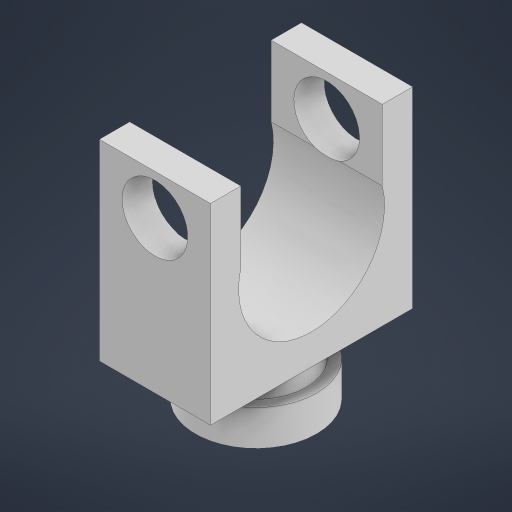
# Autodesk Inventor part: Part5
Saved by Autodesk Inventor 2023 (Build 270158030, 158C)
## iProperties
Created: 2023-02-06
Part Number: Part5
Material: Generic
Document SubType Name: Modeling
Designer: Monster
Density: 1 g/cm^3
Appearance: Default
Author: Monster
Autodesk Inventor part; units mm, degrees
ref_plane "YZ Plane" through (0, 0, 0) normal (1, 0, 0) x (0, 1, 0)
ref_plane "XZ Plane" through (0, 0, 0) normal (0, 1, 0) x (-1, 0, 0)
ref_plane "XY Plane" through (0, 0, 0) normal (0, 0, 1) x (1, 0, 0)
sketch "Sketch2" plane through (0, 0, 0) normal (0, 1, 0) x (-1, 0, 0)
  line L0 (0, 0) -> (0, -20)
  line L1 (0, -20) -> (11, -20)
  line L2 (11, -20) -> (11, 0)
  line L3 (11, 0) -> (0, 0)
  dimension "d3" = 11
  dimension "d35" = 20
  constraints: 8 end point, 3 perpendicular, 1 vertical
  measures "d3" distance of L0.end L1.end
  measures "d35" distance between parallel lines of L3 L1
extrude "Extrusion1" add sketch "Sketch2" along normal blind 15
sketch "Sketch3" plane through (-11, 0, 0) normal (0, 0, 1) x (1, 0, 0)
  line L0 (0, 0) -> (11, 0) projected
  line L1 (11, 0) -> (11, 15) projected
  line L2 (0, 15) -> (11, 15) projected
  line L3 (0, 0) -> (0, 15) projected
  line L4 (11, 15) -> (0, 15) projected
  circle A0 centre (5.5, 15) radius 3.25
  line L5 (0, 15) -> (0, 19)
  line L6 (0, 19) -> (11, 19)
  line L7 (11, 19) -> (11, 15)
  point P0 (8.75, 15)
  point P1 (2.25, 15)
  dimension "d33" = 6.5
  dimension "d34" = 4
  constraints: 6 end point, 2 perpendicular, 1 centre point, 1 midpoint, 1 vertical
  measures "d33" diameter of A0
  measures "d34" distance between parallel lines of L2 L6
extrude "Extrusion2" cut sketch "Sketch3" against normal blind 32.25 contours L2 A0 picked at (4.4481, 14.7407)
sketch "Sketch4" plane through (0, 0, 0) normal (1, 0, 0) x (0, 0, -1)
  line L0 (0, 0) -> (20, 0) projected
  line L1 (20, 0) -> (20, 15) projected
  line L2 (0, 15) -> (20, 15) projected
  line L3 (0, 0) -> (0, 15) projected
  line L4 (0, 15) -> (3, 15)
  line L5 (0, 15) -> (20, 15) projected
  line L6 (20, 15) -> (17, 15)
  line L7 (17, 15) -> (17, 12)
  line L8 (0, 11.75) -> (20, 11.75) projected
  line L9 (17, 12) -> (3, 12)
  line L10 (3, 12) -> (3, 15)
  line L11 (20, 0) -> (0, 0) projected
  line L12 (10, 0) -> (10, 3)
  arc A0 (3, 12) -> (17, 12) centre (10, 10.2222) ccw
  line L13 (3, 15) -> (3, 23.7535)
  line L14 (3, 23.7535) -> (17, 23.7535)
  line L15 (17, 23.7535) -> (17, 15)
  point P0 (17, 15)
  dimension "d11" = 3
  dimension "d12" = 3
  dimension "d36" = 3
  dimension "d37" = 3
  constraints: 18 end point, 5 perpendicular, 3 point on circle, 2 point on line, 2 vertical, 1 centre point, 1 midpoint
  measures "d11" distance of L6.end L7.end
  measures "d12" distance of L12.start L12.end
  measures "d36" distance between parallel lines of L3 L10
  measures "d37" distance between parallel lines of L1 L7
extrude "Extrusion3" cut sketch "Sketch4" against normal blind 32.25 contours A0 L8 | A0 L9 L8 | L2 L7 L9 L10
sketch "Sketch7" plane through (0, 0, 0) normal (0, -1, 0) x (1, 0, 0)
  line L0 (0, -20) -> (-11, -20) projected
  line L1 (0, 0) -> (0, -20) projected
  line L2 (-11, 0) -> (0, 0) projected
  line L3 (-11, -20) -> (-11, 0) projected
  circle A0 centre (-5.5, -10) radius 5
  line L4 (-11, -3) -> (-11, 0) projected
  line L5 (-11, 0) -> (-11, -10)
  line L6 (-11, -17.2222) -> (-11, -2.7778) projected
  line L7 (-11, -10) -> (0, -10)
  line L8 (0, -2.7778) -> (0, -17.2222) projected
  line L9 (-8.75, 0) -> (-2.25, 0) projected
  line L10 (-5.5, 0) -> (-5.5, -10)
  point P0 (-11, -17)
  point P1 (0, -17)
  point P2 (0, -3)
  dimension "d22" = 10
  dimension "d38" = 10
  constraints: 6 end point, 4 midpoint, 1 centre point
  measures "d22" diameter of A0
  measures "d38" distance of L2.start L5.end
extrude "Extrusion6" add sketch "Sketch7" along normal blind 2 contours L7 L10 A0 | A0 L7 | A0 L10 L7
sketch "Sketch8" plane through (-5.5, -2, -10) normal (0, -1, 0) x (1, 0, 0)
  circle A0 centre (0, 0) radius 6
  point P0 (5.5, 10)
  dimension "d25" = 12
  constraints: 1 centre point
  measures "d25" diameter of A0
extrude "Extrusion7" add sketch "Sketch8" along normal blind 3.5
extrude "Extrusion8" add sketch "Sketch3" against normal blind 20 contours L5 L6 L7 L2 A0
extrude "Extrusion9" cut sketch "Sketch4" against normal blind 26 contours L13 L14 L15 L2
body "Solid1"
